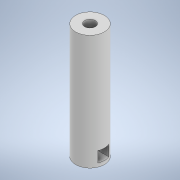
# Autodesk Inventor part: Shaft Connecting Chassis
Saved by Autodesk Inventor 2022 (Build 260153000, 153)
## iProperties
Created: 2021-12-23
Part Number: Shaft Connecting Chassis
Material: Generic
Document SubType Name: Modeling
Designer: raymo
Density: 1 g/cm^3
Appearance: Default
Author: raymo
Autodesk Inventor part; units mm, degrees
ref_plane "YZ Plane" through (0, 0, 0) normal (1, 0, 0) x (0, 1, 0)
ref_plane "XZ Plane" through (0, 0, 0) normal (0, 1, 0) x (-1, 0, 0)
ref_plane "XY Plane" through (0, 0, 0) normal (0, 0, 1) x (1, 0, 0)
sketch "Sketch1" plane through (0, 0, 0) normal (0, 1, 0) x (-1, 0, 0)
  circle A0 centre (0, 0) radius 50.8
  dimension "d0" = 101.6
  constraints: 1 centre point, 1 coincident
  measures "d0" diameter of A0
extrude "Extrusion1" add sketch "Sketch1" along normal blind 406.4
sketch "Sketch2" plane through (0, 0, 0) normal (1, 0, 0) x (0, 1, 0)
  line L0 (0, -50.8) -> (0, 50.8) projected
  line L1 (12.7, 19.05) -> (50.8, 19.05)
  line L2 (50.8, 19.05) -> (50.8, -19.05)
  line L3 (50.8, -19.05) -> (12.7, -19.05)
  line L4 (12.7, -19.05) -> (12.7, 19.05)
  point P0 (0, 0)
  dimension "d5" = 38.1
  dimension "d6" = 38.1
  constraints: 8 end point, 2 parallel, 1 horizontal, 1 perpendicular
  measures "d5" distance of L2.end L3.end
  measures "d6" distance of L1.end L2.end
extrude "Extrusion2" cut sketch "Sketch2" along normal blind 101.6
sketch "Sketch3" plane through (0, 406.4, 0) normal (0, 1, 0) x (1, 0, 0)
  circle A0 centre (0, 0) radius 19.05
  dimension "d9" = 38.1
  constraints: 1 centre point, 1 coincident
  measures "d9" diameter of A0
extrude "Extrusion3" cut sketch "Sketch3" against normal blind 393.7
body "Solid1"
